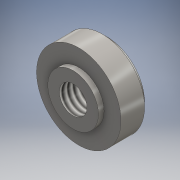
# Autodesk Inventor part: RPS Basic M3 Weld Nut
Saved by Autodesk Inventor 2016 (Build 200138000, 138)
## iProperties
Created: 2016-11-29
Part Number: RPS Basic M3 Weld Nut
Material: Stainless Steel
Document SubType Name: Modeling
Designer: R.P. SMITH
Mass: 0.813189 g
Surface Area: 1.60677 cm^2
Volume: 0.101649 cm^3
Density: 8 g/cm^3
Appearance: Semi-Polished
Author: R.P. SMITH
Autodesk Inventor part; units mm, degrees
ref_plane "YZ Plane" through (0, 0, 0) normal (1, 0, 0) x (0, 1, 0)
ref_plane "XZ Plane" through (0, 0, 0) normal (0, 1, 0) x (-1, 0, 0)
ref_plane "XY Plane" through (0, 0, 0) normal (0, 0, 1) x (1, 0, 0)
sketch "Sketch1" plane through (0, 0, 0) normal (0, 0, 1) x (1, 0, 0)
  line L0 (0, 1.5) -> (3.75, 1.5)
  line L1 (3.75, 1.5) -> (3.75, -1)
  line L2 (3.75, -1) -> (2.25, -1)
  line L3 (2.25, -1) -> (2.25, -1.5)
  line L4 (2.25, -1.5) -> (0, -1.5)
  line L5 (0, 1.5) -> (0, -1.5)
  point P0 (0, 0)
  point P1 (0, 0)
  dimension "d0" = 2.5
  dimension "d1" = 0.5
  dimension "d2" = 3.75
  dimension "d3" = 2.25
  constraints: 12 end point, 4 perpendicular, 2 coincident, 1 horizontal, 1 midpoint, 1 vertical
  measures "d0" distance of L0.end L1.end
  measures "d1" distance of L2.end L3.end
  measures "d2" distance between parallel lines of L1 L5
  measures "d3" distance of L3.end L4.end
revolve "Revolution1" add sketch "Sketch1" angle 360 about axis through (0, 1.5, 0) along (0, -1, 0)
sketch "Sketch2" plane through (0, -1.5, 0) normal (0, -1, 0) x (1, 0, 0)
  point P0 (0, 0)
  point P1 (0, 0)
  constraints: 1 coincident
hole "Hole1" at (0, -1.5, 0) direction (0, 1, 0) diameter 2.459 end through all thread size "M3x0.5" class "6H" standard "ANSI Metric M Profile"
chamfer "Chamfer1" distance 0.4 angle 45 2 edges at (0, 1.5, 1.2295) (-3.75, 1.5, 0)
body "Solid1"
